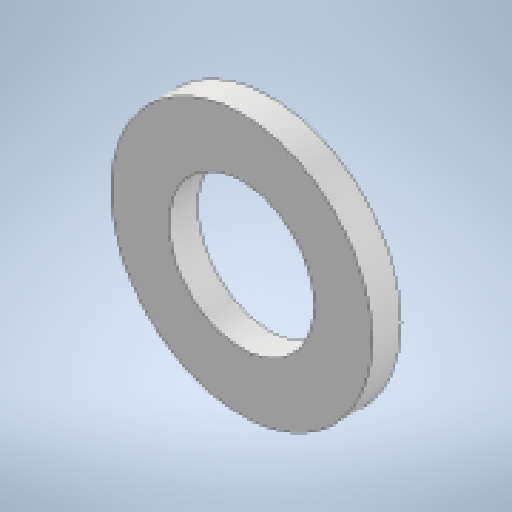
# Autodesk Inventor part: 1mm-spacer
Saved by Autodesk Inventor 2023 (Build 270158000, 158)
## iProperties
Created: 2023-01-18
Part Number: 1mm-spacer
Material: Generic
Document SubType Name: Modeling
Designer: caden
Mass: 0.0439823 g
Surface Area: 1.31947 cm^2
Volume: 0.0439823 cm^3
Density: 1 g/cm^3
Appearance: Default
Author: caden
Autodesk Inventor part; units mm, degrees
ref_plane "YZ Plane" through (0, 0, 0) normal (1, 0, 0) x (0, 1, 0)
ref_plane "XZ Plane" through (0, 0, 0) normal (0, 1, 0) x (-1, 0, 0)
ref_plane "XY Plane" through (0, 0, 0) normal (0, 0, 1) x (1, 0, 0)
sketch "Sketch1" plane through (0, 0, 0) normal (0, 0, 1) x (1, 0, 0)
  circle A0 centre (9.0271, 36.5888) radius 2.5
  circle A1 centre (9.0271, 36.5888) radius 4.5
  point P0 (0, 0)
  dimension "d0" = 5
  dimension "d1" = 9
  constraints: 2 centre point, 1 coincident
  measures "d0" diameter of A0
  measures "d1" diameter of A1
extrude "Extrusion1" add sketch "Sketch1" along normal blind 1
body "Solid1"
